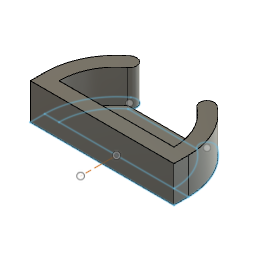
Lab3-3dprint (Autodesk Fusion 360 design; units mm, degrees)
Autodesk Fusion 360 part; units mm, degrees
sketch "Sketch1" plane through (0, 0, 0) normal (0, 1, 0) x (1, 0, 0)
  line L0 (50, 5) -> (50, -5)
  line L1 (50, -5) -> (-50, -5)
  line L2 (-50, -5) -> (-50, 5)
  line L3 (0, 5) -> (0, -20)
  line L4 (-50, 5) -> (-40, 5)
  line L5 (-40, 5) -> (0, 5)
  line L6 (40, 5) -> (50, 5)
  line L7 (0, 5) -> (40, 5)
  arc A0 (50, 5) -> (30, 45) centre (0, 5) ccw
  arc A1 (-30.0001, 45) -> (-50, 5) centre (0, 5) ccw
  arc A2 (40, 5) -> (24, 37) centre (0, 5) ccw
  arc A3 (-24, 37) -> (-40, 5) centre (0, 5) ccw
  arc A4 (-24, 37) -> (-30.0001, 45) centre (-27, 41) ccw
  line L8 (-24, 37) -> (24, 37)
  arc A5 (30, 45) -> (24, 37) centre (27, 41) ccw
  dimension "d1" = 10
  dimension "d2" = 100
  dimension "d6" = 10
  dimension "d7" = 10
  dimension "d8" = 50
  dimension "d9" = 50
  dimension "d10" = 10
  constraint horizontal L5
  constraint vertical L0
  constraint horizontal L1
  constraint vertical L2
  constraint perpendicular L1 L3
  constraint coincident L3.start L5.end
  constraint horizontal L4
  constraint tangent A2 A4
  constraint symmetric L3 A4 A5
  constraint concentric A0 A1
  constraint concentric A2 A3
  measures "d1" distance of L2.end L1.end
  measures "d2" distance of L0.end L1.end
  measures "d6" distance of L2.end L4.end
  measures "d7" distance of L0.start L6.start
  measures "d8" radius of A0
  measures "d9" radius of A0
  measures "d10" diameter of A4
extrude "Extrude1" add sketch "Sketch1" along normal blind 2 contours L5 L7 A2 A3 L8
extrude "Extrude2" add sketch "Sketch1" along normal blind 50 contours L0 L1 L3 L6 L7 | L6 A0 A2 A5 | L1 L2 L3 L4 L5 | L4 A1 A3 A4
extrude "Extrude3" cut 1 faces at (0, 50, 1.6667) along direction (0, -1, 0) blind 25
equation "d7 = d6"
equation "d10 = d6"
